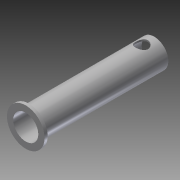
# Autodesk Inventor part: Pin
Saved by Autodesk Inventor 2013 (Build 170138000, 138)
## iProperties
Created: 2014-05-22
Part Number: Pin
Material: Steel
Document SubType Name: Modeling
Designer: nojessen
Mass: 7.25221 g
Surface Area: 28.2567 cm^2
Volume: 0.923848 cm^3
Density: 7.85 g/cm^3
Author: nojessen
Autodesk Inventor part; units mm, degrees
ref_plane "YZ Plane" through (0, 0, 0) normal (1, 0, 0) x (0, 1, 0)
ref_plane "XZ Plane" through (0, 0, 0) normal (0, 1, 0) x (-1, 0, 0)
ref_plane "XY Plane" through (0, 0, 0) normal (0, 0, 1) x (1, 0, 0)
sketch "Sketch1" plane through (0, 0, 0) normal (0, 0, 1) x (1, 0, 0)
  circle A0 centre (0, 0) radius 5.715
  circle A1 centre (0, 0) radius 5.08
  line L0 (0, 0) -> (5.715, 0)
  dimension "d0" = 11.43
  dimension "d1" = 10.16
  constraints: 2 coincident, 2 end point, 1 centre point, 1 horizontal, 1 horizontal alignment, 2 other
  measures "d1" diameter of A1
extrude "Extrusion1" add sketch "Sketch1" along normal blind 50.8
sketch "Sketch2" plane through (0, 0, 50.8) normal (0, 0, 1) x (1, 0, 0)
  circle A0 centre (0, 0) radius 5.08 projected
  circle A1 centre (0, 0) radius 5.715 projected
  circle A2 centre (0, 0) radius 7.62
  dimension "d4" = 15.24
  constraints: 1 centre point, 1 coincident
  measures "d4" diameter of A2
extrude "Extrusion2" add sketch "Sketch2" along normal blind 1.27 contours A1 | A2
ref_plane "Work Plane2" through (0, 6.35, 0) normal (0, 1, 0) x (1, 0, 0)
ref_plane "Work Plane1" through (0, 0, 0) normal (0, 1, 0) x (1, 0, 0)
sketch "Sketch3" plane through (0, 6.35, 0) normal (0, 1, 0) x (1, 0, 0)
  line L0 (0, 0) -> (0, -5.08)
  circle A0 centre (0, -5.08) radius 2.54
  dimension "d9" = 5.08
  dimension "d10" = 5.08
  constraints: 2 end point, 1 centre point, 1 coincident, 1 vertical
  measures "d9" distance of L0.start L0.end
  measures "d10" diameter of A0
extrude "Extrusion3" cut sketch "Sketch3" against normal blind 25.4
body "Solid1"
